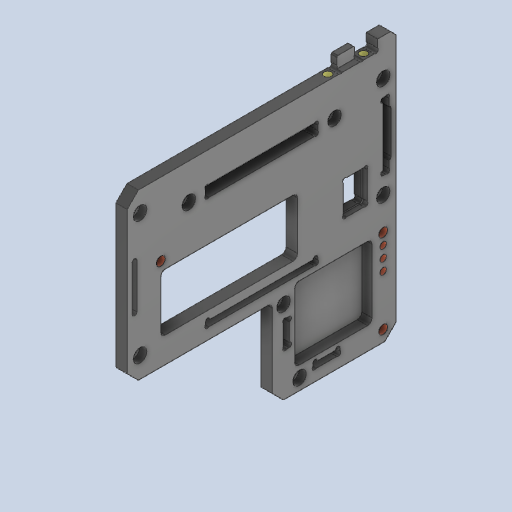
# Autodesk Inventor part: Cockpit_side_frame
Saved by Autodesk Inventor 2022 (Build 260153000, 153)
## iProperties
Part Number: Cockpit_side_frame
Material: アセタール樹脂、黒
Document SubType Name: Modeling
Designer: Masato Kubotera
Density: 1.425 g/cm^3
Appearance: 滑らか - 黒
Description: POM T5
Mass: 49.7941 g
Surface Area: 232.095 cm^2
Volume: 34.9432 cm^3
Author: Masato Kubotera
Autodesk Inventor part; units mm, degrees
ref_plane "YZ Plane" through (0, 0, 0) normal (1, 0, 0) x (0, 1, 0)
ref_plane "XZ Plane" through (0, 0, 0) normal (0, 1, 0) x (-1, 0, 0)
ref_plane "XY Plane" through (0, 0, 0) normal (0, 0, 1) x (1, 0, 0)
derived "Trunk_basis.ipt"
sketch "スケッチ1" plane through (0, 0, 0) normal (0, 1, 0) x (-1, 0, 0)
  line L0 (0, 22) -> (0, -142.9) construction
  circle A0 centre (5, 0) radius 10.5 construction
  line L1 (-7, 16) -> (36, 16) construction
  line L2 (36, 16) -> (36, -16) construction
  line L3 (36, -16) -> (-7, -16) construction
  line L4 (-7, -16) -> (-7, 16) construction
  line L5 (-7, 16) -> (36, -16) construction
  line L6 (36, 16) -> (-7, -16) construction
  line L7 (33, 13.5) -> (6, 13.5) construction
  line L8 (6, 13.5) -> (6, -13.5) construction
  line L9 (6, -13.5) -> (33, -13.5) construction
  line L10 (33, -13.5) -> (33, 13.5) construction
  line L11 (33, 13.5) -> (6, -13.5) construction
  line L12 (6, 13.5) -> (33, -13.5) construction
  line L13 (-7, 0) -> (36, 0) construction
  arc A1 (5, 16) -> (-7, 10.583) centre (5, 0) ccw construction
  line L14 (43.75, -16.25) -> (5, -16.25)
  line L15 (5, 16.25) -> (43.75, 16.25)
  line L16 (44.75, 15.25) -> (44.75, -15.25)
  arc A2 (5, 16.25) -> (-6.7376, 11.2379) centre (5, 0) ccw
  arc A3 (-6.7376, 11.2379) -> (-7.25, 9.9174) centre (-6.2711, 10.2972) ccw
  circle A4 centre (6, 13.5) radius 1.35
  line L17 (19.5, 13.5) -> (19.5, -13.5) construction
  circle A5 centre (33, 13.5) radius 1.35
  line L18 (-15, 22) -> (-20, 17)
  line L19 (-20, 17) -> (-20, -19)
  line L20 (-20, -19) -> (-28.5, -27.5)
  line L21 (-28.5, -27.5) -> (-28.5, -103)
  line L22 (57.5, -22.5) -> (57.5, 17)
  line L23 (57.5, 17) -> (52.5, 22)
  line L24 (52.5, 22) -> (-15, 22)
  line L25 (-35.5597, -116.5529) -> (-28.5, -142.9)
  line L26 (-16, -139) -> (-16, -94) construction
  line L27 (-7.5, -140.4849) -> (-7.5, -142.9)
  line L28 (-7.5, -142.9) -> (7.5, -142.9)
  line L29 (7.5, -140.4849) -> (7.5, -142.9)
  arc A6 (-7.5, -140.4849) -> (-8.9849, -139) centre (-8.2425, -139.7425) ccw
  line L30 (-17.5, -138.9955) -> (-17.5, -133) construction
  line L31 (-19, -133) -> (-16, -133) construction
  line L32 (-19, -133) -> (-19, -139) construction
  line L33 (-16, -133) -> (-16, -139) construction
  line L34 (-15, 22) -> (-10, 22) construction
  line L35 (-10, 22) -> (-10, -22) construction
  line L36 (-10, -22) -> (-15, -22) construction
  line L37 (-15, -22) -> (-15, 22) construction
  line L38 (-15, 22) -> (-10, -22) construction
  line L39 (-10, 22) -> (-15, -22) construction
  line L40 (-12.5, 22) -> (-12.5, -22) construction
  line L41 (-10, 0) -> (-15, 0) construction
  circle A7 centre (-12.5, 17.75) radius 1.6
  line L42 (-15, 10) -> (-12.5, 10) construction
  line L43 (-12.5, 10) -> (-12.5, -10) construction
  line L44 (-12.5, -10) -> (-15, -10) construction
  line L45 (-15, -10) -> (-15, 10) construction
  line L46 (-15, 10) -> (-12.5, -10) construction
  line L47 (-12.5, 10) -> (-15, -10) construction
  line L48 (-12.25, 10.25) -> (-15.25, 10.25)
  line L49 (-15.25, 8.15) -> (-15.25, -8.15)
  line L50 (-15.25, -10.25) -> (-12.25, -10.25)
  line L51 (-12.25, -8.15) -> (-12.25, 8.15)
  line L52 (-12.25, 10.25) -> (-15.25, -10.25) construction
  line L53 (-15.25, 10.25) -> (-12.25, -10.25) construction
  arc A8 (-15.25, 10.25) -> (-15.25, 8.15) centre (-15.25, 9.2) ccw
  line L54 (-13.75, 10) -> (-13.75, -10) construction
  arc A9 (-12.25, 8.15) -> (-12.25, 10.25) centre (-12.25, 9.2) ccw
  circle A10 centre (-12.5, -17.75) radius 1.6
  arc A11 (-15.25, -8.15) -> (-15.25, -10.25) centre (-15.25, -9.2) ccw
  arc A12 (-12.25, -10.25) -> (-12.25, -8.15) centre (-12.25, -9.2) ccw
  line L55 (36, 14.4) -> (44.5, 14.4) construction
  line L56 (44.5, 14.4) -> (44.5, -14.4) construction
  line L57 (36, -14.4) -> (44.5, -14.4) construction
  line L58 (49.95, 7.95) -> (49.95, -7.95)
  line L59 (52.5, 0) -> (47.5, 0) construction
  line L60 (47.5, 22) -> (52.5, 22) construction
  line L61 (52.55, -7.95) -> (52.55, 7.95)
  line L62 (51.25, 10) -> (51.25, -10) construction
  line L63 (52.5, 10) -> (50, -10) construction
  line L64 (52.5, -10) -> (50, -10) construction
  line L65 (52.5, 10) -> (52.5, -10) construction
  line L66 (50, 10) -> (52.5, -10) construction
  line L67 (49.95, -10.05) -> (52.55, -10.05)
  line L68 (49.95, 10.05) -> (52.55, -10.05) construction
  line L69 (52.55, 10.05) -> (49.95, -10.05) construction
  line L70 (52.5, -22) -> (47.5, -22) construction
  line L71 (47.5, 22) -> (52.5, -22) construction
  line L72 (52.5, 22) -> (52.5, -22) construction
  line L73 (52.5, 22) -> (47.5, -22) construction
  line L74 (50, 22) -> (50, -22) construction
  line L75 (47.5, -22) -> (47.5, 22) construction
  circle A13 centre (50, -17.75) radius 1.6
  arc A14 (52.55, -10.05) -> (52.55, -7.95) centre (52.55, -9) ccw
  line L76 (50, -10) -> (50, 10) construction
  arc A15 (49.95, -7.95) -> (49.95, -10.05) centre (49.95, -9) ccw
  arc A16 (49.95, 10.05) -> (49.95, 7.95) centre (49.95, 9) ccw
  arc A17 (52.55, 7.95) -> (52.55, 10.05) centre (52.55, 9) ccw
  line L77 (50, 10) -> (52.5, 10) construction
  line L78 (52.55, 10.05) -> (49.95, 10.05)
  circle A18 centre (50, 17.75) radius 1.6
  circle A19 centre (5, 0) radius 16 construction
  arc A20 (-6.7376, -11.2379) -> (5, -16.25) centre (5, 0) ccw
  arc A21 (-7.25, -9.9174) -> (-6.7376, -11.2379) centre (-6.2711, -10.2972) ccw
  line L79 (-7.25, -9.9174) -> (-7.25, 9.9174)
  line L80 (17.5, -138.9955) -> (17.5, -133) construction
  line L81 (19, -133) -> (19, -139) construction
  line L82 (16, -133) -> (16, -139) construction
  line L83 (19, -133) -> (16, -133) construction
  circle A22 centre (6, -13.5) radius 1.35
  circle A23 centre (33, -13.5) radius 1.35
  line L84 (-25.5, -142.9) -> (-7.5, -142.9) construction
  line L85 (25.5, -142.9) -> (7.5, -142.9) construction
  line L86 (-23.5, -22.5) -> (57.5, -22.5) construction
  line L87 (57.5, -22.5) -> (57.5, -103)
  circle A24 centre (-13.5, -55) radius 1.75
  line L88 (-11.5, -59) -> (45.5, -59)
  line L89 (47.5, -61) -> (47.5, -82.5)
  line L90 (45.5, -84.5) -> (-11.5, -84.5)
  line L91 (-13.5, -82.5) -> (-13.5, -61)
  line L92 (-13.5, -59) -> (47.5, -84.5) construction
  line L93 (47.5, -59) -> (-13.5, -84.5) construction
  line L94 (-11.5, -27.5) -> (45.5, -27.5)
  line L95 (47.5, -29.5) -> (47.5, -49)
  line L96 (45.5, -51) -> (-11.5, -51)
  line L97 (-13.5, -49) -> (-13.5, -29.5)
  line L98 (-13.5, -27.5) -> (47.5, -51) construction
  line L99 (47.5, -27.5) -> (-13.5, -51) construction
  line L100 (-23.5, -108) -> (-28.5, -103)
  circle A25 centre (-20.5415, -102) radius 1.6
  line L101 (-25.7227, -96) -> (25.7227, -96)
  line L102 (25.7227, -96) -> (34.9603, -112)
  line L103 (35.5597, -116.5529) -> (28.5, -142.9)
  line L104 (-25.7227, -96) -> (-34.9603, -112)
  line L105 (57.5, -103) -> (52.5, -108)
  arc A26 (-11.5, -27.5) -> (-13.5, -29.5) centre (-11.5, -29.5) ccw
  arc A27 (-13.5, -49) -> (-11.5, -51) centre (-11.5, -49) ccw
  arc A28 (45.5, -51) -> (47.5, -49) centre (45.5, -49) ccw
  arc A29 (47.5, -29.5) -> (45.5, -27.5) centre (45.5, -29.5) ccw
  arc A30 (-11.5, -59) -> (-13.5, -61) centre (-11.5, -61) ccw
  arc A31 (-13.5, -82.5) -> (-11.5, -84.5) centre (-11.5, -82.5) ccw
  arc A32 (45.5, -84.5) -> (47.5, -82.5) centre (45.5, -82.5) ccw
  arc A33 (47.5, -61) -> (45.5, -59) centre (45.5, -61) ccw
  line L106 (-23.5, -108) -> (52.5, -108)
  line L107 (-25.5, -139) -> (-25.5, -142.9)
  line L108 (-25.5, -142.9) -> (-28.5, -142.9)
  line L109 (-17.9813, -99.3843) -> (-16.9961, -101.0907)
  line L110 (-16.9961, -102.9093) -> (-17.9813, -104.6157)
  line L111 (-19.5563, -105.525) -> (-21.5266, -105.525)
  line L112 (-23.1016, -104.6157) -> (-24.0868, -102.9093)
  line L113 (-24.0868, -101.0907) -> (-23.1016, -99.3843)
  line L114 (-21.5266, -98.475) -> (-19.5563, -98.475)
  line L115 (-16, -94) -> (16, -94) construction
  arc A34 (-24.0868, -101.0907) -> (-24.0868, -102.9093) centre (-23.5618, -102) ccw
  arc A35 (-23.1016, -104.6157) -> (-21.5266, -105.525) centre (-22.0516, -104.6157) ccw
  arc A36 (-19.5563, -105.525) -> (-17.9813, -104.6157) centre (-19.0313, -104.6157) ccw
  arc A37 (-16.9961, -102.9093) -> (-16.9961, -101.0907) centre (-17.5211, -102) ccw
  arc A38 (-17.9813, -99.3843) -> (-19.5563, -98.475) centre (-19.0313, -99.3843) ccw
  arc A39 (-21.5266, -98.475) -> (-23.1016, -99.3843) centre (-22.0516, -99.3843) ccw
  line L116 (16, -139) -> (16, -94) construction
  line L117 (16, -94) -> (-16, -94) construction
  line L118 (-25.5, -139) -> (-8.9849, -139)
  line L119 (25.5, -142.9) -> (28.5, -142.9)
  arc A40 (8.9849, -139) -> (7.5, -140.4849) centre (8.2425, -139.7425) ccw
  circle A41 centre (29.7641, -115) radius 1.25
  line L120 (33.4891, -124.2803) -> (21.898, -121.1745) construction
  line L121 (29.7641, -115) -> (25.623, -130.4548) construction
  circle A42 centre (29.7641, -115) radius 6 construction
  circle A43 centre (-20.5415, -102) radius 6 construction
  line L122 (1.9319, -109.4824) -> (7.5588, -130.4824)
  line L123 (5.6269, -133) -> (-5.6269, -133)
  line L124 (5.3151, -110.5176) -> (10.942, -131.5176)
  line L125 (12.8739, -133) -> (17.1947, -133)
  line L126 (19.1266, -131.5176) -> (24.7535, -110.5176)
  line L127 (22.8217, -108) -> (7.2469, -108)
  circle A44 centre (25.623, -130.4548) radius 1.25
  circle A45 centre (25.623, -130.4548) radius 6 construction
  line L128 (-1.9319, -109.4824) -> (-7.5588, -130.4824)
  arc A46 (1.9319, -109.4824) -> (-1.9319, -109.4824) centre (0, -110) ccw
  arc A47 (-7.5588, -130.4824) -> (-5.6269, -133) centre (-5.6269, -131) ccw
  arc A48 (5.6269, -133) -> (7.5588, -130.4824) centre (5.6269, -131) ccw
  arc A49 (7.2469, -108) -> (5.3151, -110.5176) centre (7.2469, -110) ccw
  arc A50 (24.7535, -110.5176) -> (22.8217, -108) centre (22.8217, -110) ccw
  arc A51 (17.1947, -133) -> (19.1266, -131.5176) centre (17.1947, -131) ccw
  arc A52 (10.942, -131.5176) -> (12.8739, -133) centre (12.8739, -131) ccw
  arc A53 (-5.3151, -110.5176) -> (-7.2469, -108) centre (-7.2469, -110) ccw
  line L129 (-22.8217, -108) -> (-7.2469, -108)
  line L130 (-5.3151, -110.5176) -> (-10.942, -131.5176)
  arc A54 (-22.8217, -108) -> (-24.7535, -110.5176) centre (-22.8217, -110) ccw
  line L131 (-19.1266, -131.5176) -> (-24.7535, -110.5176)
  arc A55 (-19.1266, -131.5176) -> (-17.1947, -133) centre (-17.1947, -131) ccw
  line L132 (-12.8739, -133) -> (-17.1947, -133)
  arc A56 (-12.8739, -133) -> (-10.942, -131.5176) centre (-12.8739, -131) ccw
  circle A57 centre (-29.7641, -115) radius 1.25
  circle A58 centre (-25.623, -130.4548) radius 1.25
  arc A59 (35.5597, -116.5529) -> (34.9603, -112) centre (29.7641, -115) ccw
  arc A60 (-34.9603, -112) -> (-35.5597, -116.5529) centre (-29.7641, -115) ccw
  arc A61 (-24.0151, -139) -> (-25.5, -140.4849) centre (-24.7575, -139.7425) ccw
  line L133 (25.5, -139) -> (25.5, -142.9)
  arc A62 (25.5, -140.4849) -> (24.0151, -139) centre (24.7575, -139.7425) ccw
  line L134 (25.5, -139) -> (8.9849, -139)
  line L135 (21.5266, -98.475) -> (19.5563, -98.475)
  line L136 (16.9961, -102.9093) -> (17.9813, -104.6157)
  arc A63 (21.5266, -105.525) -> (23.1016, -104.6157) centre (22.0516, -104.6157) ccw
  circle A64 centre (20.5415, -102) radius 1.6
  line L137 (24.0868, -101.0907) -> (23.1016, -99.3843)
  arc A65 (24.0868, -102.9093) -> (24.0868, -101.0907) centre (23.5618, -102) ccw
  line L138 (23.1016, -104.6157) -> (24.0868, -102.9093)
  arc A66 (23.1016, -99.3843) -> (21.5266, -98.475) centre (22.0516, -99.3843) ccw
  line L139 (19.5563, -105.525) -> (21.5266, -105.525)
  arc A67 (19.5563, -98.475) -> (17.9813, -99.3843) centre (19.0313, -99.3843) ccw
  arc A68 (17.9813, -104.6157) -> (19.5563, -105.525) centre (19.0313, -104.6157) ccw
  line L140 (17.9813, -99.3843) -> (16.9961, -101.0907)
  arc A69 (16.9961, -101.0907) -> (16.9961, -102.9093) centre (17.5211, -102) ccw
  line L141 (16, -139) -> (16, -94) construction
  circle A70 centre (20.5415, -102) radius 6 construction
  arc A71 (29.5045, -117.5445) -> (31.2612, -117.0738) centre (30.247, -116.802) ccw construction
  line L142 (31.8379, -116.4971) -> (31.2612, -117.0738) construction
  line L143 (29.5045, -117.5445) -> (28.7167, -117.3334) construction
  arc A72 (27.4307, -116.0474) -> (28.7167, -117.3334) centre (28.4449, -116.3192) ccw construction
  line L144 (27.4307, -116.0474) -> (27.2196, -115.2596) construction
  line L145 (27.6903, -113.5029) -> (28.267, -112.9262) construction
  arc A73 (30.0237, -112.4555) -> (28.267, -112.9262) centre (29.2813, -113.198) ccw construction
  arc A74 (27.6903, -113.5029) -> (27.2196, -115.2596) centre (27.9621, -114.5171) ccw construction
  line L146 (30.0237, -112.4555) -> (30.8116, -112.6666) construction
  arc A75 (31.8379, -116.4971) -> (32.3086, -114.7404) centre (31.5662, -115.4829) ccw construction
  arc A76 (32.0975, -113.9526) -> (30.8116, -112.6666) centre (31.0833, -113.6808) ccw construction
  line L147 (32.0975, -113.9526) -> (32.3086, -114.7404) construction
  line L148 (-20.5415, -102) -> (20.5415, -102) construction
  circle A77 centre (0, -102) radius 1.6
  line L149 (0.4078, -104.525) -> (-0.4078, -104.525)
  arc A78 (-0.4078, -99.475) -> (-1.9828, -100.3843) centre (-0.9328, -100.3843) ccw
  arc A79 (0.4078, -104.525) -> (1.9828, -103.6157) centre (0.9328, -103.6157) ccw
  line L150 (2.3906, -102.9093) -> (1.9828, -103.6157)
  line L151 (-0.4078, -99.475) -> (0.4078, -99.475)
  arc A80 (1.9828, -100.3843) -> (0.4078, -99.475) centre (0.9328, -100.3843) ccw
  line L152 (1.9828, -100.3843) -> (2.3906, -101.0907)
  arc A81 (2.3906, -102.9093) -> (2.3906, -101.0907) centre (1.8656, -102) ccw
  line L153 (-2.3906, -101.0907) -> (-1.9828, -100.3843)
  arc A82 (-2.3906, -101.0907) -> (-2.3906, -102.9093) centre (-1.8656, -102) ccw
  line L154 (-1.9828, -103.6157) -> (-2.3906, -102.9093)
  arc A83 (-1.9828, -103.6157) -> (-0.4078, -104.525) centre (-0.9328, -103.6157) ccw
  circle A84 centre (0, -102) radius 1.25
  arc A85 (44.75, 15.25) -> (43.75, 16.25) centre (43.75, 15.25) ccw
  arc A86 (43.75, -16.25) -> (44.75, -15.25) centre (43.75, -15.25) ccw
  circle A87 centre (-22.75, -31.75) radius 3
  circle A88 centre (-22.75, -86.75) radius 3
  line L155 (-23.5, -96) -> (-28.5, -91) construction
  line L156 (-26, -93.5) -> (-22.75, -93.5) construction
  line L157 (-26, -25) -> (-22.75, -25) construction
  line L158 (-26, -25) -> (-26, -93.5) construction
  line L159 (-22.75, -25) -> (-22.75, -93.5) construction
  line L160 (-22.75, -59.25) -> (-28.5, -59.25) construction
  point P0 (0, 0)
  point P1 (14.5, 0)
  point P2 (19.5, 0)
  point P3 (44.75, 16.25)
  point P4 (-7.25, 10.6771)
  point P5 (19.5, 0)
  point P6 (-12.5, 0)
  point P7 (-13.75, 0)
  point P8 (44.75, 14.4)
  point P9 (44.75, -14.4)
  point P10 (51.25, 0)
  point P11 (50, 0)
  point P12 (44.75, -16.25)
  point P13 (17, -71.75)
  point P14 (17, -39.25)
  point P15 (-18.5063, -98.475)
  point P16 (-16.4711, -102)
  point P17 (-18.5063, -105.525)
  point P18 (-22.5766, -105.525)
  point P19 (-22.5766, -98.475)
  point P20 (-24.6118, -102)
  point P21 (-22.5766, -105.525)
  point P22 (-18.5063, -105.525)
  point P23 (-16.4711, -102)
  point P24 (-18.5063, -98.475)
  point P25 (-22.5766, -98.475)
  point P26 (27.6936, -122.7274)
  point P27 (0, -102.2726)
  point P28 (0, -133)
  point P29 (-7.5, -139)
  point P30 (-22.5766, -98.475)
  point P31 (18.5063, -98.475)
  point P32 (18.5063, -98.475)
  point P33 (22.5766, -105.525)
  point P34 (22.5766, -105.525)
  point P35 (24.6118, -102)
  point P36 (22.5766, -98.475)
  point P37 (22.5766, -98.475)
  point P38 (22.5766, -98.475)
  point P39 (18.5063, -105.525)
  point P40 (16.4711, -102)
  point P41 (16.4711, -102)
  point P42 (18.5063, -105.525)
  point P43 (29.7641, -115)
  point P44 (29.7641, -115)
  point P45 (30.5187, -117.8163)
  point P46 (30.5187, -117.8163)
  point P47 (27.7025, -117.0617)
  point P48 (27.7025, -117.0617)
  point P49 (31.8258, -112.9383)
  point P50 (26.9479, -114.2454)
  point P51 (29.0095, -112.1837)
  point P52 (29.0095, -112.1837)
  point P53 (31.8258, -112.9383)
  point P54 (29.0095, -112.1837)
  point P55 (32.5804, -115.7546)
  point P56 (-1.4578, -99.475)
  point P57 (-1.4578, -99.475)
  point P58 (-1.4578, -99.475)
  point P59 (1.4578, -104.525)
  point P60 (1.4578, -99.475)
  point P61 (1.4578, -99.475)
  point P62 (2.9156, -102)
  point P63 (-2.9156, -102)
  point P64 (-1.4578, -104.525)
  point P65 (-1.4578, -104.525)
sketch "スケッチ2" plane through (0, 0, 0) normal (0, 1, 0) x (-1, 0, 0)
  line L0 (-23.5, -22.5) -> (-28.5, -27.5)
  line L1 (-28.5, -27.5) -> (-28.5, -91)
  line L2 (-28.5, -91) -> (-23.5, -96)
  line L3 (-23.5, -96) -> (34.25, -96)
  line L4 (36.25, -98) -> (36.25, -131)
  line L5 (36.25, -131) -> (41.25, -136)
  line L6 (41.25, -136) -> (86.5, -136)
  line L7 (91.5, -131) -> (91.5, -20)
  line L8 (91.5, -20) -> (89, -17.5)
  line L9 (89, -17.5) -> (83.25, -17.5)
  line L10 (83.25, -17.5) -> (83.25, -21.0151)
  line L11 (81.7651, -22.5) -> (76.9849, -22.5)
  line L12 (75.5, -21.0151) -> (75.5, -17.5)
  line L13 (75.5, -17.5) -> (67.5, -17.5)
  line L14 (67.5, -17.5) -> (67.5, -21.0151)
  line L15 (66.0151, -22.5) -> (-23.5, -22.5)
  line L16 (-25.25, -25) -> (-20.25, -25) construction
  line L17 (-20.25, -25) -> (-20.25, -93.5) construction
  line L18 (-20.25, -93.5) -> (-25.25, -93.5) construction
  line L19 (-25.25, -93.5) -> (-25.25, -25) construction
  line L20 (-26, -25) -> (-25.25, -25) construction
  line L21 (-25.25, -93.5) -> (-26, -93.5) construction
  line L22 (-26, -93.5) -> (-26, -25) construction
  line L23 (-20.25, -93.5) -> (83.25, -93.5) construction
  line L24 (-20.25, -88.5) -> (83.25, -88.5) construction
  line L25 (83.25, -22.5) -> (83.25, -90.5) construction
  line L26 (83.25, -90.5) -> (88.25, -90.5) construction
  line L27 (88.25, -90.5) -> (88.25, -22.5) construction
  line L28 (83.25, -88.5) -> (83.25, -93.5) construction
  line L29 (83.25, -91) -> (88.25, -91) construction
  line L30 (88.25, -91) -> (88.25, -133.5) construction
  line L31 (83.25, -91) -> (83.25, -133.5) construction
  line L32 (83.25, -133.5) -> (88.25, -133.5) construction
  line L33 (38.75, -133.5) -> (38.75, -128.5) construction
  line L34 (38.75, -128.5) -> (38.75, -93.5) construction
  line L35 (43.75, -93.5) -> (43.75, -128.5) construction
  line L36 (38.75, -128.5) -> (43.75, -128.5) construction
  line L37 (41.25, -128.5) -> (41.25, -93.5) construction
  line L38 (38.75, -128.5) -> (82.1145, -128.5) construction
  line L39 (82.1145, -128.5) -> (82.1145, -133.5) construction
  line L40 (82.1145, -133.5) -> (38.75, -133.5) construction
  line L41 (38.75, -131) -> (82.1145, -131) construction
  line L42 (85.75, -91) -> (85.75, -133.5) construction
  circle A0 centre (85.75, -131) radius 2
  arc A1 (83.25, -128.5) -> (88.25, -128.5) centre (85.75, -131) ccw construction
  line L43 (83.25, -91) -> (-20.25, -91) construction
  line L44 (41.25, -111) -> (43.75, -111) construction
  line L45 (60.4322, -128.5) -> (60.4322, -131) construction
  line L46 (41.2, -115.5651) -> (41.2, -106.4349)
  line L47 (43.8, -107.05) -> (43.8, -114.95)
  line L48 (43.8, -117.05) -> (41.2, -104.95) construction
  line L49 (41.2, -117.05) -> (43.8, -104.95) construction
  line L50 (56.4822, -128.45) -> (64.3822, -128.45)
  line L51 (64.9973, -131.05) -> (55.8672, -131.05)
  line L52 (54.3822, -128.45) -> (66.4822, -131.05) construction
  line L53 (66.4822, -128.45) -> (54.3822, -131.05) construction
  line L54 (41.25, -105) -> (43.75, -105) construction
  line L55 (41.25, -117) -> (43.75, -117) construction
  arc A2 (42.6849, -104.95) -> (41.2, -106.4349) centre (41.9425, -105.6925) ccw
  arc A3 (43.8, -107.05) -> (43.8, -104.95) centre (43.8, -106) ccw
  arc A4 (41.2, -115.5651) -> (42.6849, -117.05) centre (41.9425, -116.3075) ccw
  arc A5 (43.8, -117.05) -> (43.8, -114.95) centre (43.8, -116) ccw
  line L56 (54.4322, -131) -> (54.4322, -128.5) construction
  line L57 (66.4322, -128.5) -> (66.4322, -131) construction
  arc A6 (54.3822, -129.5651) -> (55.8672, -131.05) centre (55.1247, -130.3075) ccw
  arc A7 (56.4822, -128.45) -> (54.3822, -128.45) centre (55.4322, -128.45) ccw
  arc A8 (64.9973, -131.05) -> (66.4822, -129.5651) centre (65.7398, -130.3075) ccw
  arc A9 (66.4822, -128.45) -> (64.3822, -128.45) centre (65.4322, -128.45) ccw
  line L58 (54.3822, -129.5651) -> (54.3822, -128.45)
  line L59 (66.4822, -128.45) -> (66.4822, -129.5651)
  line L60 (42.6849, -104.95) -> (43.8, -104.95)
  line L61 (43.8, -117.05) -> (42.6849, -117.05)
  circle A10 centre (48.4322, -131) radius 1.6
  line L62 (88.25, -22.5) -> (88.25, -17.5) construction
  line L63 (89, -17.5) -> (89, -90.5) construction
  line L64 (89, -90.5) -> (88.25, -90.5) construction
  line L65 (-13.5, -82.5) -> (-13.5, -61) projected
  arc A11 (-13.5, -82.5) -> (-11.5, -84.5) centre (-11.5, -82.5) ccw projected
  line L66 (45.5, -84.5) -> (-11.5, -84.5) projected
  arc A12 (45.5, -84.5) -> (47.5, -82.5) centre (45.5, -82.5) ccw projected
  line L67 (47.5, -61) -> (47.5, -82.5) projected
  arc A13 (47.5, -61) -> (45.5, -59) centre (45.5, -61) ccw projected
  line L68 (-11.5, -59) -> (45.5, -59) projected
  arc A14 (-11.5, -59) -> (-13.5, -61) centre (-11.5, -61) ccw projected
  line L69 (31.5, -88.5) -> (31.5, -91) construction
  line L70 (85.75, -22.5) -> (85.75, -90.5) construction
  circle A15 centre (85.75, -34) radius 1.6
  circle A16 centre (85.75, -34) radius 3
  circle A17 centre (85.75, -79) radius 1.6
  circle A18 centre (85.75, -79) radius 3
  line L71 (88.25, -22.5) -> (83.25, -22.5) construction
  arc A19 (88.25, -91) -> (83.25, -91) centre (85.75, -131) ccw construction
  circle A20 centre (48.4322, -131) radius 3
  circle A21 centre (41.25, -99) radius 1.6
  circle A22 centre (41.25, -99) radius 3
  line L72 (6.5, -88.5) -> (6.5, -91) construction
  line L73 (56.5, -88.5) -> (56.5, -91) construction
  line L74 (55.0651, -91.05) -> (7.9349, -91.05)
  line L75 (6.45, -89.5651) -> (6.45, -88.45)
  line L76 (8.55, -88.45) -> (54.45, -88.45)
  line L77 (56.55, -88.45) -> (56.55, -89.5651)
  line L78 (56.55, -91.05) -> (6.45, -88.45) construction
  line L79 (6.45, -91.05) -> (56.55, -88.45) construction
  arc A23 (8.55, -88.45) -> (6.45, -88.45) centre (7.5, -88.45) ccw
  arc A24 (6.45, -89.5651) -> (7.9349, -91.05) centre (7.1925, -90.3075) ccw
  arc A25 (56.55, -88.45) -> (54.45, -88.45) centre (55.5, -88.45) ccw
  arc A26 (55.0651, -91.05) -> (56.55, -89.5651) centre (55.8075, -90.3075) ccw
  line L80 (-20.25, -41) -> (83.25, -41) construction
  line L81 (83.25, -36) -> (-20.25, -36) construction
  line L82 (-20.25, -36) -> (-20.25, -41) construction
  line L83 (-20.25, -38.5) -> (83.25, -38.5) construction
  line L84 (31.5, -41) -> (31.5, -36) construction
  line L85 (55.0651, -35.95) -> (7.9349, -35.95)
  line L86 (7.9349, -41.05) -> (55.0651, -41.05)
  line L87 (56.55, -35.95) -> (6.45, -41.05) construction
  line L88 (6.45, -35.95) -> (55.5877, -40.952) construction
  arc A27 (7.9349, -35.95) -> (6.45, -37.4349) centre (7.1925, -36.6925) ccw
  arc A28 (6.45, -39.5651) -> (7.9349, -41.05) centre (7.1925, -40.3075) ccw
  arc A29 (56.55, -37.4349) -> (55.0651, -35.95) centre (55.8075, -36.6925) ccw
  arc A30 (55.0651, -41.05) -> (56.55, -39.5651) centre (55.8075, -40.3075) ccw
  line L89 (6.5, -41) -> (6.5, -36) construction
  line L90 (56.5, -36) -> (56.5, -41) construction
  line L91 (6.45, -37.4349) -> (6.45, -39.5651)
  line L92 (56.55, -39.5651) -> (56.55, -37.4349)
  circle A31 centre (-1, -38.5) radius 1.6
  circle A32 centre (-1, -38.5) radius 3
  circle A33 centre (64, -38.5) radius 1.6
  circle A34 centre (64, -38.5) radius 3
  line L93 (-25.25, -49.25) -> (-26, -49.25) construction
  line L94 (-25.25, -69.25) -> (-26, -69.25) construction
  line L95 (-26, -59.25) -> (-25.25, -59.25) construction
  line L96 (-22.75, -25) -> (-22.75, -93.5) construction
  arc A35 (66.0151, -22.5) -> (67.5, -21.0151) centre (66.7575, -21.7575) ccw
  arc A36 (75.5, -21.0151) -> (76.9849, -22.5) centre (76.2425, -21.7575) ccw
  line L97 (59.75, -22.5) -> (59.75, -32.5) construction
  line L98 (59.75, -32.5) -> (83.25, -32.5) construction
  line L99 (83.25, -32.5) -> (83.25, -22.5) construction
  line L100 (71.5, -17.5) -> (71.5, -32.5) construction
  line L101 (63.5, -22.5) -> (63.5, -17.5) construction
  line L102 (79.5, -22.5) -> (79.5, -17.5) construction
  circle A37 centre (-22.75, -31.75) radius 1.6
  circle A38 centre (-22.75, -31.75) radius 3
  circle A39 centre (-22.75, -86.75) radius 1.6
  circle A40 centre (-22.75, -86.75) radius 3
  line L103 (67.5, -22.5) -> (75.5, -22.5)
  line L104 (88.25, -17.5) -> (52.5, -17.5) construction
  line L105 (52.5, -17.5) -> (52.5, -22.5) construction
  circle A41 centre (85.75, -98.5) radius 1.475
  circle A42 centre (85.75, -103.5) radius 1.475
  circle A43 centre (85.75, -108.5) radius 1.475
  line L106 (48.25, -93.5) -> (78.75, -93.5)
  line L107 (80.75, -95.5) -> (80.75, -124)
  line L108 (78.75, -126) -> (48.25, -126)
  line L109 (46.25, -124) -> (46.25, -95.5)
  arc A44 (48.25, -93.5) -> (46.25, -95.5) centre (48.25, -95.5) ccw
  arc A45 (46.25, -124) -> (48.25, -126) centre (48.25, -124) ccw
  arc A46 (78.75, -126) -> (80.75, -124) centre (78.75, -124) ccw
  arc A47 (80.75, -95.5) -> (78.75, -93.5) centre (78.75, -95.5) ccw
  arc A48 (36.25, -98) -> (34.25, -96) centre (34.25, -98) ccw
  circle A49 centre (-13.5, -55) radius 1.75 projected
  circle A50 centre (-13.5, -55) radius 2
  line L110 (77.85, -78.65) -> (68.65, -78.65) construction
  line L111 (68.65, -78.65) -> (68.65, -64.85) construction
  line L112 (68.65, -64.85) -> (77.85, -64.85) construction
  line L113 (77.85, -64.85) -> (77.85, -78.65) construction
  line L114 (77.85, -78.65) -> (68.65, -64.85) construction
  line L115 (68.65, -78.65) -> (77.85, -64.85) construction
  line L116 (67.95, -64.2) -> (78.55, -64.2) construction
  line L117 (78.55, -64.2) -> (78.55, -79.3) construction
  line L118 (78.55, -79.3) -> (67.95, -79.3) construction
  line L119 (67.95, -79.3) -> (67.95, -64.2) construction
  line L120 (67.95, -64.2) -> (78.55, -79.3) construction
  line L121 (78.55, -64.2) -> (67.95, -79.3) construction
  line L122 (69.3849, -64.15) -> (77.1151, -64.15)
  line L123 (78.6, -65.6349) -> (78.6, -77.8651)
  line L124 (78.6, -79.35) -> (67.9, -64.15) construction
  line L125 (67.9, -79.35) -> (78.6, -64.15) construction
  line L126 (77.9, -78.7) -> (68.6, -64.8) construction
  line L127 (68.6, -78.7) -> (77.9, -64.8) construction
  arc A51 (69.3849, -64.15) -> (67.9, -65.6349) centre (68.6425, -64.8925) ccw
  arc A52 (70.0849, -64.8) -> (68.6, -66.2849) centre (69.3425, -65.5425) ccw
  line L128 (67.9, -71.75) -> (78.6, -71.75) construction
  line L129 (73.25, -64.15) -> (73.25, -78.7063) construction
  arc A53 (78.6, -65.6349) -> (77.1151, -64.15) centre (77.8575, -64.8925) ccw
  arc A54 (77.9, -66.2849) -> (76.4151, -64.8) centre (77.1575, -65.5425) ccw
  arc A55 (67.9, -77.8651) -> (69.3849, -79.35) centre (68.6425, -78.6075) ccw
  arc A56 (68.6, -77.2151) -> (70.0849, -78.7) centre (69.3425, -77.9575) ccw
  arc A57 (77.1151, -79.35) -> (78.6, -77.8651) centre (77.8575, -78.6075) ccw
  arc A58 (76.4151, -78.7) -> (77.9, -77.2151) centre (77.1575, -77.9575) ccw
  line L130 (70.0849, -64.8) -> (76.4151, -64.8)
  line L131 (77.9, -66.2849) -> (77.9, -77.2151)
  line L132 (67.9, -77.8651) -> (67.9, -65.6349)
  line L133 (68.6, -77.2151) -> (68.6, -66.2849)
  line L134 (76.4151, -78.7) -> (70.0849, -78.7)
  line L135 (77.1151, -79.35) -> (69.3849, -79.35)
  line L136 (-13.5, -71.75) -> (47.5, -71.75) construction
  line L137 (85.75, -56.5) -> (88.25, -56.5) construction
  line L138 (89, -54) -> (88.25, -54) construction
  line L139 (85.7, -69.45) -> (85.7, -43.55)
  line L140 (88.2835, -71.3588) -> (85.7, -41.45) construction
  line L141 (85.7, -71.55) -> (88.3, -41.45) construction
  arc A59 (85.7, -41.45) -> (85.7, -43.55) centre (85.7, -42.5) ccw
  arc A60 (88.3, -42.9349) -> (86.8151, -41.45) centre (87.5575, -42.1925) ccw
  arc A61 (85.7, -69.45) -> (85.7, -71.55) centre (85.7, -70.5) ccw
  arc A62 (86.8151, -71.55) -> (88.3, -70.0651) centre (87.5575, -70.8075) ccw
  line L142 (85.75, -41.5) -> (88.25, -41.5) construction
  line L143 (85.75, -71.5) -> (88.25, -71.5) construction
  arc A63 (89.25, -47.1801) -> (88.3, -46.1348) centre (88.2, -47.1801) ccw
  line L144 (89.25, -47.1801) -> (89.25, -65.8199)
  line L145 (88.25, -46.5) -> (89, -46.5) construction
  line L146 (88.25, -66.5) -> (89, -66.5) construction
  arc A64 (88.3, -66.8652) -> (89.25, -65.8199) centre (88.2, -65.8199) ccw
  line L147 (88.3, -42.9349) -> (88.3, -46.1348)
  line L148 (88.3, -66.8652) -> (88.3, -70.0651)
  line L149 (86.8151, -71.55) -> (85.7, -71.55)
  line L150 (85.7, -41.45) -> (86.8151, -41.45)
  line L151 (86.5, -136) -> (91.5, -131)
  arc A65 (81.7651, -22.5) -> (83.25, -21.0151) centre (82.5075, -21.7575) ccw
  circle A66 centre (85.75, -93.5) radius 2
  circle A67 centre (85.75, -93.5) radius 4 construction
  arc A68 (-24.15, -49.25) -> (-26.25, -49.25) centre (-25.2, -49.25) ccw
  line L152 (-26, -49.25) -> (-26.25, -49.25) construction
  line L153 (-26.25, -49.25) -> (-26.25, -69.25)
  line L154 (-24.15, -49.25) -> (-24.15, -69.25)
  arc A69 (-26.25, -69.25) -> (-24.15, -69.25) centre (-25.2, -69.25) ccw
  point P0 (0, 0)
  point P1 (-25.7227, -96)
  point P2 (-23.5, -22.5)
  point P3 (42.5, -111)
  point P4 (60.4322, -129.75)
  point P5 (31.5, -89.75)
  point P6 (31.5, -38.5)
  point P7 (6.45, -41.05)
  point P8 (52.5, -22)
  point P9 (73.25, -71.75)
  point P10 (73.25, -71.75)
  point P11 (87, -56.5)
  dimension "d1" = 120
  dimension "d2" = 5
  dimension "d3" = 0.75
  dimension "d9" = 8
  dimension "d11" = 5
  dimension "d12" = 68.5
  dimension "d13" = 5
  dimension "d14" = 5
  dimension "d15" = 5
  dimension "d16" = 2.5
  dimension "d18" = 2.5
  dimension "d19" = 4
  dimension "d20" = 0.1
  dimension "d21" = 35
  dimension "d22" = 39.5
  dimension "d24" = 2.5
  dimension "d25" = 5
  dimension "d26" = 12
  dimension "d28" = 0.05
  dimension "d29" = 1.05
  dimension "d30" = 1.05
  dimension "d31" = 12
  dimension "d32" = 0.05
  dimension "d34" = 1.05
  dimension "d35" = 1.05
  dimension "d36" = 0.05
  dimension "d37" = 0.05
  dimension "d38" = 3.2
  dimension "d39" = 0.75
  dimension "d40" = 5
  dimension "d41" = 3.2
  dimension "d42" = 6
  dimension "d43" = 45
  dimension "d44" = 0.4219
  dimension "d45" = 6
  dimension "d46" = 3.2
  dimension "d47" = 6
  dimension "d48" = 24
  dimension "d49" = 50
  dimension "d50" = 1.05
  dimension "d51" = 1.05
  dimension "d52" = 0.05
  dimension "d53" = 0.05
  dimension "d54" = 5
  dimension "d55" = 13.5
  dimension "d56" = 1.05
  dimension "d57" = 50
  dimension "d58" = 0.05
  dimension "d61" = 0.05
  dimension "d62" = 73
  dimension "d63" = 3.2
  dimension "d64" = 6
  dimension "d65" = 65
  dimension "d66" = 20
  dimension "d68" = 1.05
  dimension "d69" = 10
  dimension "d70" = 23.5
  dimension "d71" = 39
  dimension "d72" = 20
  dimension "d73" = 16
  dimension "d82" = 0.5
  dimension "d83" = 3.2
  dimension "d84" = 6
  dimension "d85" = 55
  constraints: 301 end point, 107 point on circle, 101 point on line, 65 centre point, 58 midpoint, 56 symmetric about line, 53 perpendicular, 33 parallel, 16 horizontal, 13 coincident, 13 tangent, 11 vertical, 7 collinear, 3 equal radius, 49 other
  measures "d1" distance between parallel lines of L1 L7
  measures "d2" distance of L16.start L16.end
  measures "d3" distance of L20.start L20.end
  measures "d9" distance of L12.end L13.end
  measures "d11" horizontal distance of L2.end L1.end
  measures "d12" distance of L21.end L20.start
  measures "d13" distance of L34.end L35.start
  measures "d14" distance of L33.start L33.end
  measures "d15" distance of L31.end L30.end
  measures "d16" distance between parallel lines of L6 L40
  measures "d18" distance between parallel lines of L33 L4
  measures "d19" diameter of A0
  measures "d20" distance edge to line of A1 L39
  measures "d21" distance of L35.start L35.end
  measures "d22" distance between parallel lines of L31 L35
  measures "d24" distance between parallel lines of L3 L23
  measures "d25" distance of L24.end L23.end
  measures "d26" distance of L55.end L54.end
  measures "d28" distance between parallel lines of L47 L35
  measures "d29" radius of A2
  measures "d30" radius of A3
  measures "d31" distance between parallel lines of L57 L56
  measures "d32" distance between parallel lines of L50 L38
  measures "d34" radius of A7
  measures "d35" radius of A6
  measures "d36" distance between parallel lines of L58 L56
  measures "d37" distance between parallel lines of L60 L54
  measures "d38" diameter of A10
  measures "d39" distance of L63.end L26.end
  measures "d40" distance of L27.end L62.end
  measures "d41" diameter of A15
  measures "d42" diameter of A16
  measures "d43" distance of A18.centre A15.centre
  measures "d44" distance edge to line of A19 L26
  measures "d45" diameter of A20
  measures "d46" diameter of A21
  measures "d47" diameter of A22
  measures "d48" diameter of A22.centre L44
  measures "d49" distance between parallel lines of L73 L72
  measures "d50" radius of A23
  measures "d51" radius of A24
  measures "d52" distance between parallel lines of L24 L76
  measures "d53" distance between parallel lines of L72 L75
  measures "d54" distance between parallel lines of L80 L81
  measures "d55" distance between parallel lines of L81 L71
  measures "d56" radius of A27
  measures "d57" distance between parallel lines of L89 L90
  measures "d58" distance between parallel lines of L85 L81
  measures "d61" distance between parallel lines of L91 L89
  measures "d62" distance of L63.end L8.end
  measures "d63" diameter of A31
  measures "d64" diameter of A32
  measures "d65" distance of A34.centre A31.centre
  measures "d66" distance between parallel lines of L94 L93
  measures "d68" radius of A35
  measures "d69" distance of L98.end L99.end
  measures "d70" distance of L97.end L98.end
  measures "d71" distance from line of L7 point (52.5, -22)
  measures "d72" distance between parallel lines of L7 L100
  measures "d73" distance between parallel lines of L102 L101
  measures "d82" distance between parallel lines of L29 L26
  measures "d83" diameter of A37
  measures "d84" diameter of A38
  measures "d85" distance of A39.centre A37.centre
extrude "押し出し1" add sketch "スケッチ2" along normal blind 5 contours L15 A35 L103 A36 L11 A65 L10 L9 L8 L7 L151 L6 L5 L4 A48 L3 L2 L1 L0
extrude "押し出し2" add sketch "スケッチ2" along normal blind 2.5 contours A35 L14 L13 L12 A36 L103
extrude "押し出し3" add sketch "スケッチ2" along normal blind 1.9 contours A16 | A18 | A20 | A22 | A32 | A34 | A38 | A40
extrude "押し出し4" add sketch "スケッチ2" along normal blind 0.5 contours L106 A47 L107 A46 L108 A45 L109 A44
extrude "押し出し5" add sketch "スケッチ2" along normal blind 3 contours L122 A53 L123 A57 L135 A55 L132 A51
sketch "スケッチ3" plane through (-83.25, 0, -22.5) normal (0, 0, 1) x (1, 0, 0)
  line L0 (1.4849, 5) -> (6.2651, 5) projected
  line L1 (3.75, 5) -> (3.75, 0)
  line L2 (17.2349, 5) -> (106.75, 5) projected
  line L3 (19.75, 5) -> (19.75, 0)
  line L4 (1.4849, 0) -> (6.2651, 0) projected
  point P0 (83.25, 0)
  point P1 (0, 5)
  point P2 (19.75, 0)
  point P3 (0, 0)
  point P4 (3.75, 2.5)
  point P5 (19.75, 2.5)
  constraints: 4 end point, 2 midpoint, 2 point on line, 2 vertical, 1 coincident
hole "穴1" at (-79.5, 2.5, -22.5) at (-63.5, 2.5, -22.5) direction (0, 0, -1) diameter 3.4587 depth 4 thread size "M4x0.5" class "6H" standard "ISO Metric profile"
chamfer "面取り1" distance 0.5 angle 45 2 edges at (-75.5, 1.25, -17.5) (-67.5, 1.25, -17.5)
